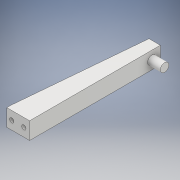
# Autodesk Inventor part: soporteAgarre
Saved by Autodesk Inventor 2017 (Build 210142000, 142)
## iProperties
Part Number: soporteAgarre
Material: Genérico
Document SubType Name: Modeling
Designer: rober
Density: 1 g/cm^3
Appearance: Valor por defecto
Author: rober
Autodesk Inventor part; units mm, degrees
ref_plane "YZ Plane" through (0, 0, 0) normal (1, 0, 0) x (0, 1, 0)
ref_plane "XZ Plane" through (0, 0, 0) normal (0, 1, 0) x (-1, 0, 0)
ref_plane "XY Plane" through (0, 0, 0) normal (0, 0, 1) x (1, 0, 0)
sketch "Boceto1" plane through (0, 0, 0) normal (0, 0, 1) x (1, 0, 0)
  line L0 (0, 0) -> (1.6, 0)
  line L1 (1.6, 0) -> (1.6, 0.3)
  line L2 (0, 0.3) -> (0, 0)
  line L3 (1.6, 0.3) -> (1.6, 8.287)
  line L4 (1.6, 8.287) -> (2.5, 8.287)
  line L5 (2.5, 8.287) -> (2.5, 8.887)
  line L6 (2.5, 8.887) -> (1.6, 8.887)
  line L7 (1.6, 8.887) -> (1.6, 9.187)
  line L8 (1.6, 9.187) -> (0.8, 9.187)
  line L9 (0.8, 9.187) -> (0, 0.3)
  line L10 (1.6, 8.887) -> (1.6, 8.287)
  constraints: 22 end point, 1 collinear
extrude "Extrusión1" add sketch "Boceto1" along normal blind 0.15 contours L2 L9 L8 L7 L10 L3 L1 L0
sketch "Boceto2" plane through (1.6, 0, 0) normal (1, 0, 0) x (0, 0, -1)
  line L0 (0, 0.3) -> (0, 9.187)
  line L1 (-1.2, 9.187) -> (-1.2, 0.3)
  line L2 (-1.2, 0.3) -> (0, 0.3)
  line L3 (-1.05, 0.3) -> (-1.05, 9.187)
  line L4 (-0.15, 0.3) -> (-0.15, 9.187)
  line L5 (-1.2, 0) -> (0, 0)
  line L6 (-1.2, 0) -> (-1.2, 0.3)
  line L7 (0, 0) -> (0, 0.3)
  line L8 (0, 9.187) -> (-1.2, 9.187)
  point P0 (0, 0)
  constraints: 18 end point, 4 point on line
extrude "Extrusión2" add sketch "Boceto2" against normal blind 0.15 contours L7 L5 L6 L2 | L2 L3 L8 L4 | L2 L1 L8 L3
sketch "Boceto3" plane through (1.6, 0, 1.2) normal (0, 0, 1) x (1, 0, 0)
  line L0 (-1.6, 0) -> (0, 0)
  line L1 (0, 0) -> (0, 0.3)
  line L2 (-1.6, 0.3) -> (-1.6, 0)
  line L3 (0, 0.3) -> (0, 8.287)
  line L4 (0, 8.287) -> (0.9, 8.287)
  line L5 (0.9, 8.287) -> (0.9, 8.887)
  line L6 (0.9, 8.887) -> (0, 8.887)
  line L7 (0, 8.887) -> (0, 9.187)
  line L8 (0, 9.187) -> (-0.8, 9.187)
  line L9 (-0.8, 9.187) -> (-1.6, 0.3)
  line L10 (0, 8.887) -> (0, 8.287)
  line L11 (0, 0) -> (-0.15, 0) projected
  point P0 (-1.6, 0)
  constraints: 22 end point, 1 vertical
extrude "Extrusión3" add sketch "Boceto3" against normal blind 0.15 contours L2 L9 L8 L7 L10 L3 L1 L0
sketch "Boceto4" plane through (1.45, 0, 0) normal (-1, 0, 0) x (0, 0, 1)
  line L0 (1.2, 0.3) -> (1.2, 9.187)
  line L1 (0, 9.187) -> (0, 0.3)
  line L2 (0, 0.3) -> (1.2, 0.3)
  line L3 (0.15, 0.3) -> (0.15, 9.187)
  line L4 (1.05, 0.3) -> (1.05, 9.187)
  line L5 (0, 0) -> (1.2, 0)
  line L6 (0, 0) -> (0, 0.3)
  line L7 (1.2, 0) -> (1.2, 0.3)
  line L8 (1.2, 9.187) -> (0, 9.187)
  point P0 (0, 0)
  constraints: 18 end point, 4 point on line
extrude "Extrusión4" add sketch "Boceto4" along normal blind 1.45 contours L7 L5 L6 L2
sketch "Boceto5" plane through (1.45, 0.3, 1.05) normal (0, 1, 0) x (1, 0, 0)
  line L0 (-1.45, 1.05) -> (0.15, 1.05)
  line L1 (0.15, 1.05) -> (0.15, -0.15)
  line L2 (0.15, -0.15) -> (-1.45, -0.15)
  line L3 (-1.45, -0.15) -> (-1.45, 1.05)
  circle A0 centre (-1.1, 0.45) radius 0.15
  circle A1 centre (-0.25, 0.45) radius 0.15
  line L4 (0.15, 0.15) -> (1.05, 0.15)
  line L5 (1.05, 0.15) -> (1.05, 0.75)
  line L6 (1.05, 0.75) -> (0.15, 0.75)
  line L7 (0, 1.05) -> (0, -0.15)
  line L8 (0.15, 1.05) -> (0.15, -0.15) projected
  point P0 (-1.45, 1.05)
  constraints: 16 end point, 4 point on line, 2 centre point
extrude "Extrusión5" cut sketch "Boceto5" against normal blind 1.45 contours A0 | A1
sketch "Boceto6" plane through (1.6, 0, 0) normal (1, 0, 0) x (0, 0, -1)
  line L0 (0, 0) -> (-1.2, 0) projected
  line L1 (0, 0) -> (0, 9.187) projected
  line L2 (0, 9.187) -> (-1.2, 9.187) projected
  line L3 (-1.2, 9.187) -> (-1.2, 0) projected
  line L4 (0, 0.3) -> (0, 9.187)
  line L5 (-1.2, 9.187) -> (-1.2, 0.3)
  line L6 (-1.2, 0) -> (0, 0)
  line L7 (-1.2, 0) -> (-1.2, 0.3)
  line L8 (0, 0) -> (0, 0.3)
  line L9 (0, 9.187) -> (-1.2, 9.187)
  circle A0 centre (-0.6, 8.587) radius 0.3
  constraints: 12 end point, 1 centre point
extrude "Extrusión6" add sketch "Boceto6" along normal blind 0.9 contours A0
